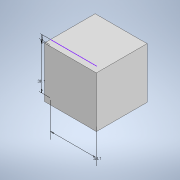
# Autodesk Inventor part: cornerbracket1
Saved by Autodesk Inventor 2020 (Build 240168000, 168)
## iProperties
Created: 2021-02-21
Part Number: cornerbracket1
Material: Generic
Document SubType Name: Modeling
Designer: AOB
Mass: 24.0032 g
Surface Area: 108.268 cm^2
Volume: 24.0032 cm^3
Density: 1 g/cm^3
Appearance: Default
Author: AOB
Autodesk Inventor part; units mm, degrees
ref_plane "YZ Plane" through (0, 0, 0) normal (1, 0, 0) x (0, 1, 0)
ref_plane "XZ Plane" through (0, 0, 0) normal (0, 1, 0) x (-1, 0, 0)
ref_plane "XY Plane" through (0, 0, 0) normal (0, 0, 1) x (1, 0, 0)
sketch "Sketch1" plane through (0, 0, 0) normal (0, 0, 1) x (1, 0, 0)
  line L0 (38.1, 0) -> (38.1, -38.1)
  line L1 (38.1, -38.1) -> (0, -38.1)
  line L2 (0, -38.1) -> (0, 0)
  line L3 (0, -1) -> (0, 4)
  line L4 (0, 4) -> (38.1, 4)
  line L5 (38.1, 4) -> (38.1, 0)
  line L6 (38.1, -1) -> (0, -1)
  dimension "d0" = 38.1
  dimension "d1" = 38.1
  dimension "d2" = 5
  constraints: 14 end point, 3 perpendicular, 2 point on line, 1 parallel, 1 vertical
  measures "d0" distance of L1.end L2.end
  measures "d1" distance of L0.end L1.end
  measures "d2" distance of L3.start L3.end
extrude "Extrusion1" add sketch "Sketch1" along normal blind 5
extrude "Extrusion2" add sketch "Sketch1" against normal blind 37.1 contours L0 L6 L2 L3 L4 L5
sketch "Sketch2" plane through (38.1, -38.1, 5) normal (1, 0, 0) x (0, 0, -1)
  line L0 (0, 42.1) -> (42.2269, 42.1)
  line L1 (42.2269, 42.1) -> (42.2269, -0.127)
  line L2 (42.2269, -0.127) -> (0, -0.127)
  line L3 (0, -0.127) -> (0, 42.1)
  point P0 (5, 38.1)
  dimension "d7" = 42.227
  dimension "d8" = 42.2269
  constraints: 8 end point, 2 parallel, 1 horizontal, 1 perpendicular
  measures "d7" distance of L0.end L1.end
  measures "d8" distance of L1.end L2.end
extrude "Extrusion3" add sketch "Sketch2" along normal blind 5
body "Solid1"
